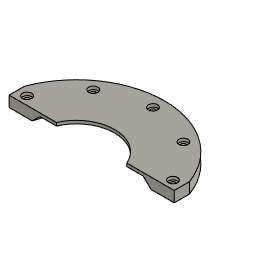
BasementBase v5 (Autodesk Fusion 360 design; units mm, degrees)
Autodesk Fusion 360 part; units mm, degrees
sketch "Sketch1" plane through (0, 0, 0) normal (0, 0, 1) x (1, 0, 0)
  circle A0 centre (0, 50) radius 1.6
  circle A1 centre (0, 0) radius 40
  line L0 (0, 0) -> (0, 50) construction
  circle A2 centre (-47.5528, 15.4509) radius 1.6
  line L1 (53.8012, 10.0063) -> (53.8006, 20.0063)
  arc A3 (53.8006, 20.0063) -> (-53.803, 20) centre (0, 0) ccw
  circle A4 centre (47.5528, 15.4509) radius 1.6
  circle A5 centre (-29.3893, 40.4508) radius 1.6
  circle A6 centre (29.3893, 40.4508) radius 1.6
  line L2 (-53.803, 20) -> (-53.8024, 10)
  line L3 (-53.8024, 10) -> (53.8012, 10.0063)
  circle A7 centre (0, 0) radius 50 construction
  line L4 (-53.8024, 10) -> (-53.8018, 0) construction
  line L5 (-53.8018, 0) -> (0, 0) construction
  circle A8 centre (0, 0) radius 25
  circle A9 centre (-47.5528, 15.4509) radius 3
  circle A10 centre (-29.3893, 40.4508) radius 3
  circle A11 centre (0, 50) radius 3
  circle A12 centre (29.3893, 40.4508) radius 3
  circle A13 centre (47.5528, 15.4509) radius 3
  dimension "d268" = 3.2
  dimension "d13" = 80
  dimension "d14" = 57.4
  dimension "d16" = 30.9017
  dimension "d17" = 30.9017
  dimension "d18" = 30.9017
  dimension "d19" = 30.9017
  dimension "d20" = 10
  dimension "d21" = 10
  dimension "d22" = 100
  dimension "d23" = 3.2
  dimension "d24" = 3.2
  dimension "d25" = 3.2
  dimension "d26" = 3.2
  dimension "d32" = 50
  dimension "d33" = 6
  dimension "d34" = 6
  dimension "d35" = 6
  dimension "d36" = 6
  dimension "d37" = 6
  constraint coincident A1.centre L0.start
  constraint coincident A0.centre L0.end
  constraint coincident L2 L3.start
  constraint coincident L1 L3.end
  constraint perpendicular L1 L3
  constraint coincident A0.centre A7
  constraint vertical L0
  constraint perpendicular L2 L3
  constraint equal L1 L2
  constraint coincident L1.start L3.end
  constraint coincident A2.centre A7
  constraint coincident A5.centre A7
  constraint coincident A6.centre A7
  constraint coincident A4.centre A7
  constraint perpendicular L3 L4
  constraint perpendicular L0 L5
  constraint concentric A4 A13
  constraint coincident A2.centre A9.centre
  constraint coincident A5.centre A10.centre
  constraint coincident A6.centre A12.centre
  measures "d268" diameter of A0
  measures "d13" diameter of A1
  measures "d14" radius of A3
  measures "d16" distance of A5.centre A0.centre
  measures "d17" distance of A5.centre A2.centre
  measures "d18" distance of A0.centre A6.centre
  measures "d19" distance of A4.centre A6.centre
  measures "d20" distance of A3.end L2.end
  measures "d21" distance of L2.end L4.end
  measures "d22" diameter of A7
  measures "d23" diameter of A2
  measures "d24" diameter of A5
  measures "d25" diameter of A6
  measures "d26" diameter of A4
  measures "d32" diameter of A8
  measures "d33" diameter of A9
  measures "d34" diameter of A10
  measures "d35" diameter of A11
  measures "d36" diameter of A12
  measures "d37" diameter of A13
extrude "Extrude1" add sketch "Sketch1" against normal blind 5 contours A1 L1 A3 L2 L3 | A9 | A10 | A11 | A12 | A13
extrude "Extrude2" add sketch "Sketch1" along normal blind 2 contours A1 L3 A8 | A1 L1 A3 L2 L3 picked at (-31.3201, 15.4348)
chamfer "Chamfer1" distance 5 angle 45 1 edges at (-0.0024, 40, 0)
